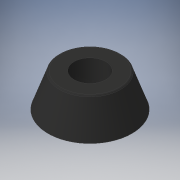
# Autodesk Inventor part: BushingTop
Saved by Autodesk Inventor 2019 (Build 230136000, 136)
## iProperties
Created: 2020-12-10
Part Number: BushingTop
Material: Rubber, Black
Document SubType Name: Modeling
Designer: Anass Hamdi
Density: 0.93 g/cm^3
Appearance: Rubber - Black
Author: Anass Hamdi
Autodesk Inventor part; units mm, degrees
ref_plane "YZ Plane" through (0, 0, 0) normal (1, 0, 0) x (0, 1, 0)
ref_plane "XZ Plane" through (0, 0, 0) normal (0, 1, 0) x (-1, 0, 0)
ref_plane "XY Plane" through (0, 0, 0) normal (0, 0, 1) x (1, 0, 0)
sketch "Sketch1" plane through (0, 0, 0) normal (0, 0, 1) x (1, 0, 0)
  line L0 (-4.7, 0) -> (-12.5, 0)
  line L1 (0, 0) -> (0, 10) construction
  line L2 (-4.7, 10) -> (-9, 10)
  line L3 (-9, 10) -> (-12.5, 0)
  line L4 (-4.7, 10) -> (-4.7, 0)
  dimension "d0" = 12.5
  dimension "d1" = 10
  dimension "d4" = 4.7
  dimension "d5" = 9
  constraints: 10 end point, 2 horizontal, 1 perpendicular, 1 vertical
  measures "d0" distance of L1.start L0.end
  measures "d1" distance of L1.start L1.end
  measures "d4" distance of L1.end L2.start
  measures "d5" distance of L1.end L2.end
revolve "Revolution1" add sketch "Sketch1" angle 360 about axis through (0, 0, 0) along (0, 1, 0)
fillet "Fillet1" radius 0.5 1 edges at (9, 10, 0)
body "Solid1"
